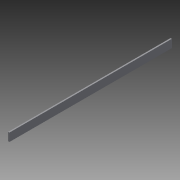
# Autodesk Inventor part: Mirroir
Saved by Autodesk Inventor 2015 SP1 (Build 190203100, 203)
## iProperties
Created: 2015-03-28
Part Number: Mirroir
Material: Generic
Document SubType Name: Modeling
Designer: Cyril
Density: 1 g/cm^3
Appearance: Default
Author: Cyril
Autodesk Inventor part; units mm, degrees
ref_plane "YZ Plane" through (0, 0, 0) normal (1, 0, 0) x (0, 1, 0)
ref_plane "XZ Plane" through (0, 0, 0) normal (0, 1, 0) x (-1, 0, 0)
ref_plane "XY Plane" through (0, 0, 0) normal (0, 0, 1) x (1, 0, 0)
sketch "Sketch1" plane through (0, 0, 0) normal (0, 0, 1) x (1, 0, 0)
  line L0 (-8, -50) -> (8, -50)
  line L1 (8, -50) -> (8, 50)
  line L2 (8, 50) -> (-8, 50)
  line L3 (-8, 50) -> (-8, -50)
  line L4 (-8, -50) -> (8, 50) construction
  line L5 (8, -50) -> (-8, 50) construction
  point P0 (0, 0)
  dimension "d0" = 100
  dimension "d1" = 16
  constraints: 12 end point, 2 midpoint, 2 parallel, 1 horizontal, 1 perpendicular
  measures "d0" distance of L2.end L0.start
  measures "d1" distance of L1.end L2.end
extrude "Extrusion1" add sketch "Sketch1" along normal mid plane 2000
body "Solid1"
